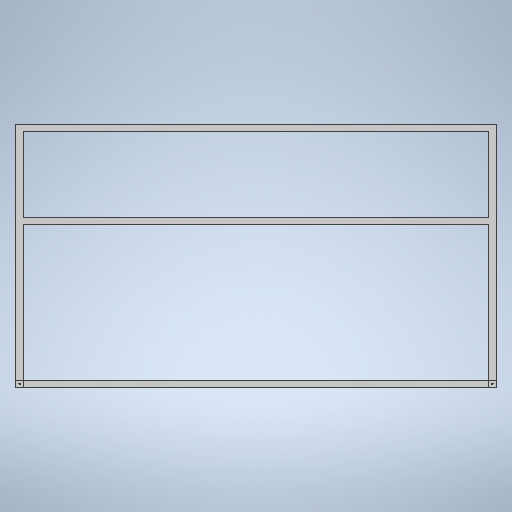
# Autodesk Inventor part: Frame of Monitor Mount
Saved by Autodesk Inventor 2027 (Build 310192000, 192)
## iProperties
Created: 2026-05-21
Part Number: Frame of Monitor Mount
Material: Generic
Document SubType Name: Modeling
Designer: IG2
Density: 1 g/cm^3
Appearance: Default
Author: IG2
Autodesk Inventor part; units mm, degrees
ref_plane "YZ Plane" through (0, 0, 0) normal (1, 0, 0) x (0, 1, 0)
ref_plane "XZ Plane" through (0, 0, 0) normal (0, 1, 0) x (-1, 0, 0)
ref_plane "XY Plane" through (0, 0, 0) normal (0, 0, 1) x (1, 0, 0)
sketch "Sketch1" plane through (0, 0, 0) normal (0, 0, 1) x (1, 0, 0)
  line L0 (0, 0) -> (-508, 0)
  line L1 (-508, 0) -> (0, 0)
  line L2 (0, 0) -> (508, 0)
  line L3 (508, 0) -> (508, 25.4)
  line L4 (508, 25.4) -> (-508, 25.4)
  line L5 (-508, 25.4) -> (-508, 0)
  dimension "d2" = 508
  dimension "d3" = 25.4
  dimension "d190" = 1016
  constraints: 12 end point, 2 horizontal, 2 perpendicular, 1 collinear, 1 parallel
  measures "d2" distance of L0.start L2.end
  measures "d3" distance of L2.end L3.end
  measures "d190" distance of L3.end L4.end
extrude "Right Base Leg" add sketch "Sketch1" along normal blind 25.4
sketch "Sketch2" plane through (0, 0, 25.4) normal (0, 0, 1) x (1, 0, 0)
  line L0 (0, 0) -> (-12.7, 0)
  line L1 (-508, 0) -> (508, 0) projected
  line L2 (0, 0) -> (12.7, 0) construction
  line L3 (-12.7, 0) -> (-12.7, 25.4)
  line L4 (-12.7, 25.4) -> (12.7, 25.4)
  line L5 (12.7, 25.4) -> (12.7, 0)
  line L6 (12.7, 0) -> (0, 0)
  dimension "d7" = 12.7
  dimension "d8" = 180
  dimension "d9" = 25.4
  dimension "d10" = 25.4
  constraints: 12 end point, 2 collinear, 1 horizontal, 1 perpendicular, 1 vertical
  measures "d7" distance of L0.start L0.end
  measures "d8" angle of L0 L2
  measures "d9" distance of L0.end L3.end
  measures "d10" distance of L3.end L4.end
extrude "Base Leg Connection" add sketch "Sketch2" along normal blind 1524
sketch "Sketch3" plane through (0, 0, 1549.4) normal (0, 0, 1) x (1, 0, 0)
  line L0 (-508, 0) -> (-12.7, 0) projected
  line L1 (0, 0) -> (-508, 0)
  line L2 (-508, 0) -> (-508, 25.4)
  line L3 (508, 0) -> (508, 25.4) projected
  line L4 (508, 0) -> (508, 25.4)
  line L5 (-508, 25.4) -> (508, 25.4)
  line L6 (508, 25.4) -> (508, 0)
  line L7 (508, 0) -> (0, 0)
  point P0 (-12.7, 0)
  dimension "d13" = 508
  dimension "d14" = 25.4
  dimension "d15" = 25.4
  constraints: 12 end point, 2 perpendicular, 2 vertical, 1 collinear
  measures "d13" distance of L1.start L0.start
  measures "d14" distance of L0.start L2.end
  measures "d15" distance of L3.end L3.start
extrude "Left Base Leg" add sketch "Sketch3" along normal blind 25.4
sketch "Sketch5" plane through (-508, 25.4, 0) normal (0, 1, 0) x (1, 0, 0)
  line L0 (520.7, -25.4) -> (1016, -25.4) projected
  line L1 (520.7, -25.4) -> (520.7, 0)
  line L2 (520.7, -25.4) -> (495.3, -25.4)
  line L3 (495.3, -25.4) -> (495.3, 0)
  line L4 (495.3, 0) -> (520.7, 0)
  point P0 (508, 0)
  constraints: 8 end point, 2 perpendicular, 1 vertical
extrude "Right Side Beam" add sketch "Sketch5" along normal blind 838.2
sketch "Sketch6" plane through (-508, 25.4, 1549.4) normal (0, 1, 0) x (1, 0, 0)
  line L0 (520.7, 1524) -> (520.7, 0) projected
  line L1 (520.7, 0) -> (520.7, -25.4)
  line L2 (495.3, 1524) -> (495.3, 0) projected
  line L3 (520.7, 0) -> (495.3, 0)
  line L4 (495.3, 0) -> (495.3, -25.4)
  line L5 (1016, -25.4) -> (0, -25.4) projected
  line L6 (495.3, -25.4) -> (520.7, -25.4)
  point P0 (508, 1549.4)
  point P1 (520.7, -25.4)
  constraints: 8 end point, 1 collinear, 1 horizontal, 1 perpendicular, 1 point on line, 1 vertical
extrude "Left Side Beam" add sketch "Sketch6" along normal blind 838.2
sketch "Sketch8" plane through (12.7, 25.4, 25.4) normal (0, 0, 1) x (1, 0, 0)
  line L0 (-25.4, 0) -> (-25.4, 838.2) projected
  line L1 (-25.4, 838.2) -> (-25.4, 812.8)
  line L2 (-25.4, 812.8) -> (-25.4, 838.2)
  line L3 (-25.4, 838.2) -> (0, 838.2)
  line L4 (0, 838.2) -> (0, 812.8)
  line L5 (0, 812.8) -> (-25.4, 812.8)
  point P0 (-12.7, -25.4)
  dimension "d22" = 25.4
  dimension "d23" = 25.4
  dimension "d24" = 25.4
  constraints: 10 end point, 3 perpendicular, 1 collinear, 1 point on line
  measures "d22" distance of L0.end L1.end
  measures "d23" distance of L1.end L0.end
  measures "d24" distance of L0.end L3.end
extrude "Top Beam" add sketch "Sketch8" along normal blind 1524
sketch "Sketch9" plane through (12.7, 0, 1549.4) normal (1, 0, 0) x (0, 0, -1)
  line L0 (0, 0) -> (61.2151, 0)
  line L1 (0, 25.4) -> (0, 863.6) projected
  line L2 (0, 533.4) -> (1524, 533.4)
  line L3 (1524, 0) -> (0, 0) projected
  line L4 (0, 533.4) -> (0, 558.8)
  line L5 (0, 558.8) -> (1524, 558.8)
  line L6 (1524, 558.8) -> (1524, 533.4)
  point P0 (1549.4, 0)
  point P1 (0, 838.2)
  point P2 (762, 533.4)
  dimension "d27" = 533.4
  dimension "d29" = 25.4
  dimension "d30" = 1524
  dimension "d31" = 90
  constraints: 10 end point, 2 horizontal, 2 point on line, 1 midpoint, 1 parallel, 1 perpendicular
  measures "d27" distance from line of point (762, 533.4) L3
  measures "d29" distance of L2.start L4.end
  measures "d30" distance of L4.end L5.end
  measures "d31" angle of L4 L5
extrude "First Middle Beam" add sketch "Sketch9" against normal blind 25.4
sketch "Sketch10" plane through (12.7, 25.4, 0) normal (1, 0, 0) x (0, 0, -1)
  line L0 (-1549.4, 0) -> (-1549.4, 508) projected
  line L1 (-1549.4, 508) -> (-1168.4, 508)
  line L2 (-1549.4, 508) -> (-1168.4, 508) construction
  line L3 (-1168.4, 508) -> (-787.4, 508)
  line L4 (-787.4, 508) -> (-406.4, 508)
  line L5 (-1549.4, 508) -> (-25.4, 508) projected
  line L6 (-406.4, 508) -> (-25.4, 508)
  line L7 (-1168.4, 508) -> (-1181.1, 508)
  line L8 (-25.4, 533.4) -> (-1549.4, 533.4) projected
  line L9 (-1181.1, 533.4) -> (-1155.7, 533.4)
  point P0 (0, -25.4)
  dimension "d34" = 381
  dimension "d36" = 381
  dimension "d37" = 381
  constraints: 14 end point, 4 point on line, 3 collinear, 2 horizontal
  measures "d34" distance of L0.end L1.end
  measures "d36" distance of L1.end L3.end
  measures "d37" distance of L3.end L4.end
sketch "Sketch11" plane through (12.7, 558.8, 1549.4) normal (0, 1, 0) x (1, 0, 0)
  point P0 (-12.7, 1549.4)
sketch "Sketch19" plane through (508, 0, 0) normal (1, 0, 0) x (0, 0, -1)
  line L0 (-25.4, 0) -> (-25.4, 25.4) projected
  line L1 (0, 25.4) -> (-25.4, 25.4) projected
  point P0 (0, 0)
  point P1 (-12.7, 12.7)
  dimension "d82" = 12.7
  dimension "d83" = 12.7
  measures "d82" distance from line of L0 point (-12.7, 12.7)
  measures "d83" distance from line of point (-12.7, 12.7) L1
hole "Hole for Right Side Beam on Base" at (508, 12.7, 12.7) direction (-1, 0, 0) diameter 5.08 end through all
sketch "Sketch20" plane through (-508, 0, 1549.4) normal (-1, 0, 0) x (0, 0, 1)
  line L0 (0, 25.4) -> (25.4, 25.4) projected
  line L1 (0, 25.4) -> (0, 0) projected
  point P0 (-1549.4, 0)
  point P1 (12.7, 12.7)
  dimension "d91" = 12.7
  dimension "d92" = 12.7
  measures "d91" distance from line of L0 point (12.7, 12.7)
  measures "d92" distance from line of L1 point (12.7, 12.7)
hole "Hole for Left Side Beam on Base" at (-508, 12.7, 1562.1) direction (1, 0, 0) diameter 5.08 end through all
sketch "Sketch23" plane through (-508, 863.6, 0) normal (0, 1, 0) x (1, 0, 0)
  line L0 (520.7, -1574.8) -> (520.7, 0) projected
  line L1 (495.3, -1574.8) -> (520.7, -1574.8) projected
  point P0 (508, 0)
  point P1 (508, -1562.1)
  dimension "d119" = 12.7
  dimension "d120" = 12.7
  measures "d119" distance from line of L0 point (508, -1562.1)
  measures "d120" distance from line of L1 point (508, -1562.1)
hole "Hole3" at (0, 863.6, 1562.1) direction (0, -1, 0) diameter 5.08 end through all
sketch "Sketch24" plane through (-508, 863.6, 0) normal (0, 1, 0) x (1, 0, 0)
  line L0 (495.3, 0) -> (495.3, -1574.8) projected
  line L1 (520.7, 0) -> (495.3, 0) projected
  point P0 (508, 0)
  point P1 (508, -12.7)
  dimension "d128" = 12.7
  dimension "d129" = 12.7
  measures "d128" distance from line of L0 point (508, -12.7)
  measures "d129" distance from line of L1 point (508, -12.7)
hole "Hole4" at (0, 863.6, 12.7) direction (0, -1, 0) diameter 5.08 end through all
sketch "Sketch25" plane through (0, 0, 0) normal (0, 0, -1) x (-1, 0, 0)
  line L0 (-12.7, 25.4) -> (-12.7, 863.6) projected
  line L1 (12.7, 25.4) -> (508, 25.4) projected
  point P0 (0, 0)
  point P1 (0, 12.7)
  point P2 (-12.7, 820.6966)
  dimension "d137" = 12.7
  dimension "d138" = 12.7
  measures "d137" distance from line of L0 point (0, 12.7)
  measures "d138" distance from line of L1 point (0, 12.7)
hole "Hole5" at (0, 12.7, 0) direction (0, 0, 1) diameter 5.08 end through all
sketch "Sketch26" plane through (0, 0, 1574.8) normal (0, 0, 1) x (1, 0, 0)
  point P0 (0, 0)
  point P1 (-0.9051, 1619.5448)
hole "Hole6" [suppressed]
sketch "Sketch28" plane through (0, 0, 0) normal (0, 0, -1) x (-1, 0, 0)
  line L0 (12.7, 558.8) -> (-12.7, 558.8) projected
  line L1 (-12.7, 25.4) -> (-12.7, 863.6) projected
  point P0 (0, 0)
  point P1 (0, 546.1)
  point P2 (-12.7, 871.4966)
  dimension "d162" = 12.7
  dimension "d163" = 12.7
  measures "d162" distance from line of point (0, 546.1) L0
  measures "d163" distance from line of L1 point (0, 546.1)
hole "Hole8" at (0, 546.1, 0) direction (0, 0, 1) diameter 5.08 end through all
sketch "Sketch29" plane through (-508, 863.6, 0) normal (0, 1, 0) x (1, 0, 0)
  line L0 (901.7, -1181.0938) -> (927.1, -1181.1) projected
  line L1 (520.7, -1574.8) -> (520.7, 0) projected
  point P0 (508, 0)
  point P1 (508, -1168.2982)
  point P2 (520.7, 0)
  dimension "d171" = 12.7
  dimension "d172" = 12.7
  constraints: 1 other
  measures "d171" distance from line of point (508, -1168.298) L0
hole "Hole9" [suppressed]
sketch "Sketch30" plane through (-508, 863.6, 0) normal (0, 1, 0) x (1, 0, 0)
  line L0 (927.1, -774.7) -> (901.7, -774.7) projected
  line L1 (495.3, 0) -> (495.3, -1574.8) projected
  point P0 (508, 0)
  point P1 (508, -787.4)
  point P2 (495.3, -1574.8)
  dimension "d180" = 12.7
  dimension "d181" = 12.7
  constraints: 1 other
  measures "d180" distance from line of L0 point (508, -787.4)
hole "Hole10" [suppressed]
sketch "Sketch31" plane through (-508, 863.6, 0) normal (0, 1, 0) x (1, 0, 0)
  line L0 (495.3, 0) -> (495.3, -1574.8) projected
  point P0 (508, 0)
  point P1 (508, -406.6756)
  dimension "d189" = 12.7
  measures "d189" distance from line of L0 point (508, -406.676)
hole "Hole11" at (0, 863.6, 406.6756) direction (0, -1, 0) diameter 5.08 end through all
body "Solid1"
